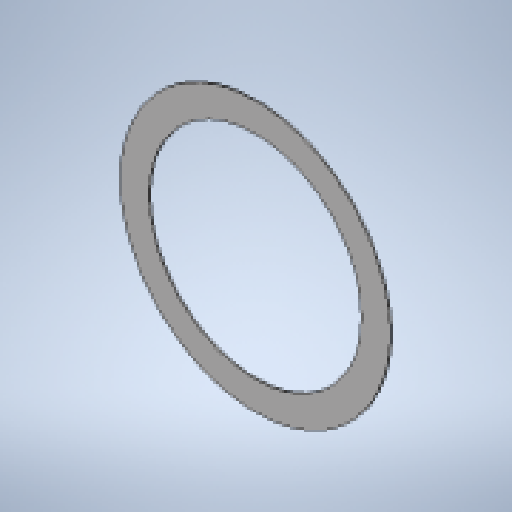
# Autodesk Inventor part: DMF2.0 01 45 Gear ring 5
Saved by Autodesk Inventor 2025.3 (Build 293356030, 356C)
## iProperties
Created: 2024-04-30
Part Number: DMF2.0 01 45 Gear ring 5
Material: Generic
Document SubType Name: Sheet Metal
Designer: admin
Stock Number: Барабан_Сектор_Усилителя
Density: 1 g/cm^3
Sheet Metal Rule: Default
Sheet Metal Width: 0,000 mm
Sheet Metal Length: 0,000 mm
Sheet Metal Area: 0,000 mm^2
Appearance: Default
Author: pokla
Autodesk Inventor part; units mm, degrees
ref_plane "YZ Plane" through (0, 0, 0) normal (1, 0, 0) x (0, 1, 0)
ref_plane "XZ Plane" through (0, 0, 0) normal (0, 1, 0) x (-1, 0, 0)
ref_plane "XY Plane" through (0, 0, 0) normal (0, 0, 1) x (1, 0, 0)
sketch "Sketch1" plane through (0, 0, 0) normal (0, 0, 1) x (1, 0, 0)
  circle A0 centre (0, 0) radius 125
  circle A1 centre (0, 0) radius 175
  dimension "d31" = 350
  dimension "d32" = 250
  measures "d31" diameter of A1
  measures "d32" diameter of A0
extrude "Plate1" add sketch "Sketch1" against normal blind 2
equation "\"d15\" = Thickness"
equation "\"BendRadius\" = Thickness"
equation "\"BendReliefWidth\" = Thickness"
equation "\"BendReliefDepth\" = 0.5 * Thickness"
equation "\"CornerReliefSize\" = 4 * Thickness"
equation "\"MinimumRemnant\" = 2 * Thickness"
equation "\"TransitionRadius\" = BendRadius"
equation "\"JacobiRadiusSize\" = BendRadius"
equation "\"GapSize\" = Thickness"
equation "\"Thickness\" = 2"
body "Solid1"
